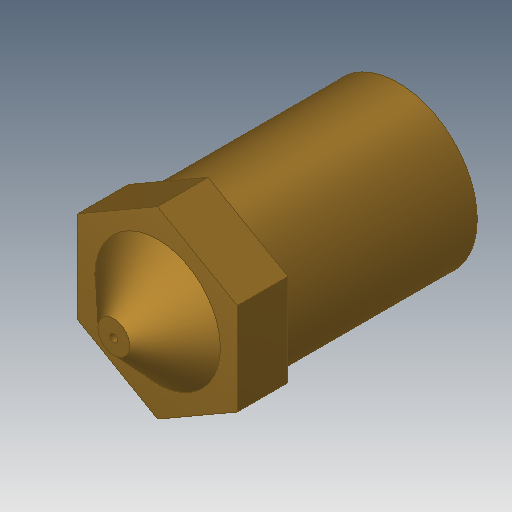
# Autodesk Inventor part: nozzel
Saved by Autodesk Inventor 2019 (Build 230136000, 136)
## iProperties
Created: 2018-11-13
Part Number: nozzel
Material: Brass, Soft Yellow
Document SubType Name: Modeling
Designer: LillaHunden
Density: 8.47 g/cm^3
Appearance: Brass - Satin
Mass: 3.84648 g
Surface Area: 5.82788 cm^2
Volume: 0.45413 cm^3
Author: LillaHunden
Autodesk Inventor part; units mm, degrees
ref_plane "YZ Plane" through (0, 0, 0) normal (1, 0, 0) x (0, 1, 0)
ref_plane "XZ Plane" through (0, 0, 0) normal (0, 1, 0) x (-1, 0, 0)
ref_plane "XY Plane" through (0, 0, 0) normal (0, 0, 1) x (1, 0, 0)
sketch "Sketch1" plane through (0, 0, 0) normal (0, 0, 1) x (1, 0, 0)
  circle A0 centre (0, 0) radius 3.965
  dimension "d0" = 7.93
  constraints: 1 centre point, 1 coincident
  measures "d0" diameter of A0
extrude "Extrusion1" add sketch "Sketch1" along normal blind 9.54
sketch "Sketch2" plane through (0, 0, 9.54) normal (0, 0, 1) x (1, 0, 0)
  circle A0 centre (0, 0) radius 3.965 projected
  line L0 (0, 4.6188) -> (4, 2.3094)
  line L1 (4, 2.3094) -> (4, -2.3094)
  line L2 (4, -2.3094) -> (0, -4.6188)
  line L3 (0, -4.6188) -> (-4, -2.3094)
  line L4 (-4, -2.3094) -> (-4, 2.3094)
  line L5 (-4, 2.3094) -> (0, 4.6188)
  dimension "d4" = 8
  constraints: 12 end point, 1 coincident, 13 other
  measures "d4" distance between parallel lines of L4 L1
extrude "Extrusion2" add sketch "Sketch2" along normal blind 2.54 contours A0 | L0 L1 L2 L3 L4 L5
ref_plane "Work Plane1" through (0, -2.3094, 9.54) normal (1, 0, 0) x (0, 0, -1)
sketch "Sketch3" plane through (0, -2.3094, 9.54) normal (1, 0, 0) x (0, 0, -1)
  line L0 (-2.54, 2.3576) -> (-4.74, 2.3576)
  line L1 (-4.74, 3.1576) -> (-2.54, 5.5076)
  line L2 (-4.74, 3.1576) -> (-4.74, 2.3576)
  line L3 (-2.54, 0) -> (-2.54, 4.6188) projected
  line L4 (9.54, 2.3094) -> (2.1715, 2.3094)
  line L5 (-2.54, 4.6188) -> (-2.54, 6.9282) projected
  line L6 (-2.54, 5.5076) -> (-2.54, 2.3576)
  point P0 (-2.54, 2.3094)
  dimension "d7" = 3.15
  dimension "d9" = 2.2
  dimension "d10" = 0.8
  constraints: 10 end point, 3 point on line, 2 horizontal, 1 collinear, 1 horizontal alignment, 1 midpoint, 1 perpendicular, 1 vertical alignment
  measures "d7" distance of L1.end L0.start
  measures "d9" distance of L0.start L0.end
  measures "d10" distance of L1.start L0.end
revolve "Revolution1" add sketch "Sketch3" angle 360 about axis through (0, 0.0482, 12.08) along (0, 0, 1)
sketch "Sketch4" plane through (0, 0.0482, 14.28) normal (0, 0, 1) x (1, 0, 0)
  circle A0 centre (0, -0.0482) radius 0.2
  dimension "d12" = 0.4
  constraints: 1 centre point, 1 coincident
  measures "d12" diameter of A0
extrude "Extrusion3" cut sketch "Sketch4" against normal through all
sketch "Sketch5" plane through (0, 0, 0) normal (0, 0, -1) x (-1, 0, 0)
  circle A0 centre (0, 0) radius 0.2 projected
  circle A1 centre (0, 0) radius 2.55
  point P0 (0, 0)
  dimension "d15" = 5.1
  constraints: 1 centre point, 1 coincident
  measures "d15" diameter of A1
extrude "Extrusion4" cut sketch "Sketch5" against normal blind 9.17 contours A0 | A1
thread "Thread1" size "M5.5x0.5" class "6H" standard "ANSI Metric M Profile" full length
body "Solid1"
